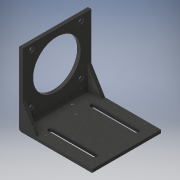
# Autodesk Inventor part: NEMA23_StepperonlineMount
Saved by Autodesk Inventor 2019.4 (Build 234330000, 330)
## iProperties
Created: 2021-01-26
Part Number: NEMA23_StepperonlineMount
Material: Generic
Document SubType Name: Modeling
Designer: Jorian Brusind
Density: 1 g/cm^3
Appearance: Fine Textured - Black
Author: Jorian Brusind
Autodesk Inventor part; units mm, degrees
ref_plane "YZ Plane" through (0, 0, 0) normal (1, 0, 0) x (0, 1, 0)
ref_plane "XZ Plane" through (0, 0, 0) normal (0, 1, 0) x (-1, 0, 0)
ref_plane "XY Plane" through (0, 0, 0) normal (0, 0, 1) x (1, 0, 0)
sketch "Sketch1" plane through (0, 0, 0) normal (0, 1, 0) x (-1, 0, 0)
  line L0 (0, 0) -> (69, 0)
  line L1 (69, 0) -> (69, -65)
  line L2 (69, -65) -> (0, -65)
  line L3 (0, -65) -> (0, 0)
  dimension "d0" = 69
  dimension "d1" = 65
  constraints: 8 end point, 2 parallel, 1 horizontal, 1 perpendicular
  measures "d0" distance of L1.end L2.end
  measures "d1" distance of L0.end L1.end
extrude "Extrusion1" add sketch "Sketch1" along normal blind 3
sketch "Sketch2" plane through (0, 3, 0) normal (0, 1, 0) x (1, 0, 0)
  line L0 (0, 65) -> (-69, 65) projected
  line L1 (-69, 65) -> (-66, 65)
  line L2 (-66, 65) -> (-66, 0)
  line L3 (-66, 0) -> (-69, 0)
  line L4 (-69, 0) -> (-69, 65)
  point P0 (0, 0)
  dimension "d4" = 3
  dimension "d5" = 65
  constraints: 8 end point, 2 parallel, 1 horizontal, 1 perpendicular
  measures "d4" distance of L2.end L3.end
  measures "d5" distance of L1.end L2.end
extrude "Extrusion2" add sketch "Sketch2" along normal blind 66
fillet "Fillet1" radius 2 2 edges at (-66, 3, -32.5) (-69, 0, -32.5)
sketch "Sketch3" plane through (0, 0, 0) normal (0, 0, 1) x (1, 0, 0)
  line L0 (-67, 0) -> (0, 0) projected
  line L1 (-66, 0) -> (-51, 0) construction
  line L2 (-66, 5) -> (-66, 69) projected
  line L3 (-66, 5) -> (-66, 0)
  line L4 (-66, 5) -> (-61, 5) construction
  line L5 (-66, 0) -> (-51, 0)
  line L6 (-66, 0) -> (-66, 25)
  line L7 (-66, 25) -> (-51, 0)
  dimension "d12" = 5
  dimension "d13" = 90
  dimension "d14" = 15
  dimension "d15" = 90
  dimension "d16" = 25
  constraints: 12 end point, 3 perpendicular, 2 horizontal, 1 point on line
  measures "d12" distance of L2.start L1.start
  measures "d13" angle of L3 L4
  measures "d14" distance of L1.start L1.end
  measures "d15" angle of L5 L3
  measures "d16" distance of L1.start L6.end
extrude "Extrusion3" add sketch "Sketch3" against normal blind 3
pattern_linear "Rectangular Pattern1" count 2 spacing 62 along (0, 0, -1) of "Extrusion3"
sketch "Sketch4" plane through (-66, 69, 0) normal (1, 0, 0) x (0, 0, -1)
  circle A0 centre (32.5, -29) radius 22.5
  line L0 (0, 0) -> (65, 0) projected
  line L1 (0, -44) -> (0, 0) projected
  point P0 (0, -69)
  dimension "d22" = 45
  dimension "d23" = 29
  dimension "d24" = 32.5
  constraints: 1 centre point
  measures "d22" diameter of A0
  measures "d23" distance from line of L0 A0.centre
  measures "d24" distance from line of L1 A0.centre
extrude "Extrusion4" cut sketch "Sketch4" against normal blind 3
sketch "Sketch5" plane through (-66, 69, 0) normal (1, 0, 0) x (0, 0, -1)
  circle A0 centre (9, -5.501) radius 2.6
  line L0 (0, 0) -> (65, 0) projected
  line L1 (0, -44) -> (0, 0) projected
  circle A1 centre (56, -5.501) radius 2.6
  circle A2 centre (9, -52.501) radius 2.6
  circle A3 centre (56, -52.501) radius 2.6
  point P0 (0, -69)
  dimension "d27" = 5.2
  dimension "d28" = 5.501
  dimension "d29" = 9
  dimension "d32" = 47
  dimension "d35" = 47
  constraints: 4 centre point, 1 horizontal, 1 vertical, 6 other
  measures "d27" diameter of A0
  measures "d28" distance from line of L0 A0.centre
  measures "d29" distance from line of L1 A0.centre
  measures "d32" distance of A0.centre A1.centre
  measures "d35" distance of A0.centre A2.centre
extrude "Extrusion5" cut sketch "Sketch5" against normal blind 3
sketch "Sketch6" plane through (0, 3, 0) normal (0, 1, 0) x (1, 0, 0)
  line L0 (-52.8, 0) -> (0, 0) projected
  line L1 (0, 0) -> (0, 65) projected
  arc A0 (-10, 10.4) -> (-10, 14.6) centre (-10, 12.5) ccw
  arc A1 (-52, 14.6) -> (-52, 10.4) centre (-52, 12.5) ccw
  line L2 (-10, 14.6) -> (-52, 14.6)
  line L3 (-69, 65) -> (-69, 0) projected
  line L4 (-10, 12.5) -> (-7.9, 12.5) construction
  line L5 (-10, 10.4) -> (-52, 10.4)
  dimension "d47" = 4.2
  dimension "d48" = 4.2
  dimension "d49" = 12.5
  dimension "d50" = 12.5
  dimension "d52" = 42
  dimension "d54" = 17
  constraints: 6 end point, 4 point on circle, 2 centre point, 1 horizontal, 1 tangent
  measures "d47" diameter of A0
  measures "d48" diameter of A1
  measures "d49" distance from line of L0 L4.start
  measures "d50" distance from line of L0 A1.centre
  measures "d52" distance of L2.start L2.end
  measures "d54" distance from line of L3 A1.centre
extrude "Extrusion6" cut sketch "Sketch6" against normal blind 3
pattern_linear "Rectangular Pattern2" count 2 spacing 40 along (0, 0, -1) of "Extrusion6"
body "Solid1"
